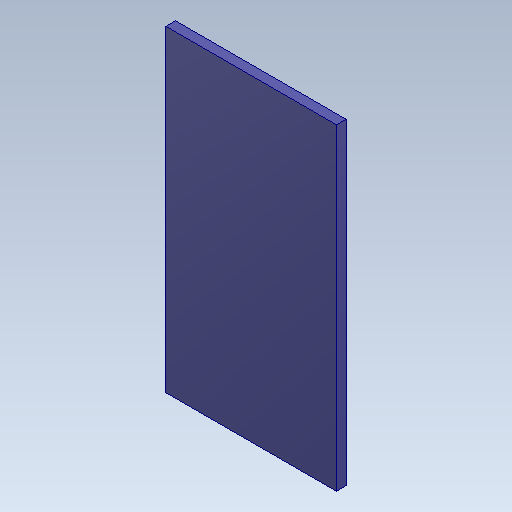
# Autodesk Inventor part: ARDUINO1_ARDUINO_PRO_MINI
Saved by Autodesk Inventor 2020 (Build 240168000, 168)
## iProperties
Created: 2019-08-29
Part Number: ARDUINO1_ARDUINO_PRO_MINI
Material: Generic
Document SubType Name: Modeling
Designer: psrob
Density: 1 g/cm^3
Appearance: ARDUINO_PRO_MINI, ARDUINO1_ARDUINO_PRO_MINI
Author: psrob
Autodesk Inventor part; units mm, degrees
ref_plane "YZ Plane" through (0, 0, 0) normal (1, 0, 0) x (0, 1, 0)
ref_plane "XZ Plane" through (0, 0, 0) normal (0, 1, 0) x (-1, 0, 0)
ref_plane "XY Plane" through (0, 0, 0) normal (0, 0, 1) x (1, 0, 0)
sketch "ARDUINO_PRO_MINI, ARDUINO1_ARDUINO_PRO_MINI_1" plane through (0, 0, 0) normal (0, 0, 1) x (1, 0, 0)
  line L0 (-5.08, 12.7) -> (12.7, 12.7)
  line L1 (12.7, 12.7) -> (12.7, -20.3835)
  line L2 (12.7, -20.3835) -> (-5.08, -20.3835)
  line L3 (-5.08, -20.3835) -> (-5.08, 12.7)
  constraints: 8 end point
extrude "Extrusion1" add sketch "ARDUINO_PRO_MINI, ARDUINO1_ARDUINO_PRO_MINI_1" along normal blind 1
body "Solid1"
